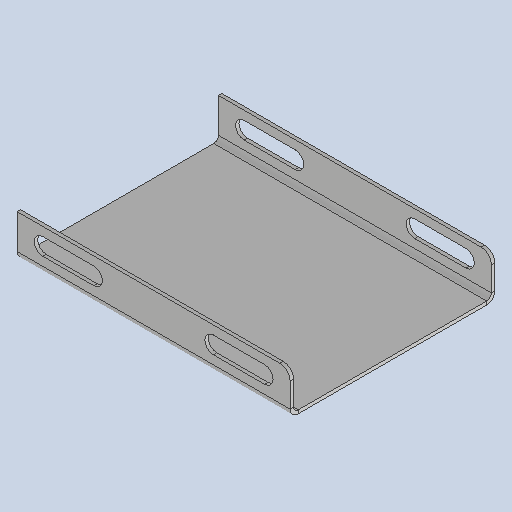
# Autodesk Inventor part: TRM 026 right board damper
Saved by Autodesk Inventor 2025 (Build 290162010, 162A)
## iProperties
Created: 2024-08-07
Part Number: TRM 026 right board damper
Material: AISI 304
Document SubType Name: Sheet Metal
Designer: pokla
Density: 8.02768 g/cm^3
Flat Pattern Width: 16.2404 cm
Flat Pattern Length: 16 cm
Flat Pattern Area: 259.846 cm^2
Sheet Metal Rule: AISI304 2mm Die16
Sheet Metal Width: 162.404 mm
Sheet Metal Length: 160.000 mm
Sheet Metal Area: 25984.637 mm^2
Appearance: Default
Stock Number: ТРМ 026 правый борт успокоитель
Mass: 393.603 g
Surface Area: 510.428 cm^2
Volume: 49.0307 cm^3
Author: pokla
Autodesk Inventor part; units mm, degrees
note: some values were not read from the file. Chosen so that the rebuilt part matches the saved one: flange form of "Plate2".
ref_plane "YZ Plane" through (0, 0, 0) normal (1, 0, 0) x (0, 1, 0)
ref_plane "XZ Plane" through (0, 0, 0) normal (0, 1, 0) x (-1, 0, 0)
ref_plane "XY Plane" through (0, 0, 0) normal (0, 0, 1) x (1, 0, 0)
sketch "Sketch1" plane through (0, 0, 0) normal (0, 0, 1) x (1, 0, 0)
  line L0 (-80, -60) -> (80, -60)
  line L1 (80, -60) -> (80, 60)
  line L2 (80, 60) -> (-80, 60)
  line L3 (-80, 60) -> (-80, -60)
  line L4 (-80, -60) -> (80, 60) construction
  line L5 (80, -60) -> (-80, 60) construction
  point P0 (0, 0)
  dimension "d0" = 160
  dimension "d1" = 120
  measures "d0" distance of L2.end L1.end
  measures "d1" distance of L1.end L0.end
extrude "Plate1" add sketch "Sketch1" along normal blind 2
sketch "Sketch2" plane through (0, 0, 0) normal (0, 0, -1) x (-1, 0, 0)
  line L0 (-60, 40) -> (140, 40) construction
  line L1 (140, 40) -> (140, 20) construction
  line L2 (140, 20) -> (-60, 20) construction
  line L3 (-60, 20) -> (-60, 40) construction
  line L4 (-80, 60) -> (80, 60) projected
  line L5 (-80, -60) -> (-80, 60) projected
  point P0 (0, 0)
  point P1 (-48, 100)
  point P2 (-50, 98)
  dimension "d6" = 200
  dimension "d9" = 20
  dimension "d10" = 20
  dimension "d11" = 20
  constraints: 4 other
  measures "d6" distance of L0.start L0.end
  measures "d9" distance of L0.end L1.end
  measures "d11" length of L3
mark "Mark1"
sketch "Sketch3" plane through (80, 58, 0) normal (0, 1, 0) x (-1, 0, 0)
  line L0 (160, 0) -> (0, 0)
  line L1 (0, 0) -> (0, -25)
  line L2 (0, -25) -> (160, -25)
  line L3 (160, -25) -> (160, 0)
  constraints: 6 end point, 1 horizontal, 1 perpendicular, 1 vertical
edge flange "Flange1" height 25 angle 90 thickness 2 bend radius 2.75 thickness toward (0, 1, 0) relief round relief width 2 relief depth 1 corner gap 2.75 corner form 0 edges at (0, 60, 0) (0, -60, 0) wall of the first edge with corners at (-80, 58, 0) (80, 58, 0) (80, 58, 25) (-80, 58, 25)
bend "Bend1"
corner "Corner1"
sketch "Sketch4" plane through (0, 0, 0) normal (0, 1, 0) x (-1, 0, 0)
  line L0 (-80, 4.75) -> (80, 4.75) construction
  line L1 (80, 4.75) -> (80, 25) projected
  line L2 (80, 25) -> (-80, 25) construction
  line L3 (-80, 4.75) -> (-80, 25) projected
  line L4 (-65, 14.875) -> (-35, 14.875) construction
  line L5 (-65, 9.875) -> (-35, 9.875)
  line L6 (-35, 19.875) -> (-65, 19.875)
  arc A0 (-65, 19.875) -> (-65, 9.875) centre (-65, 14.875) ccw
  arc A1 (-35, 9.875) -> (-35, 19.875) centre (-35, 14.875) ccw
  line L7 (35, 14.875) -> (65, 14.875) construction
  line L8 (35, 9.875) -> (65, 9.875)
  line L9 (65, 19.875) -> (35, 19.875)
  arc A2 (35, 19.875) -> (35, 9.875) centre (35, 14.875) ccw
  arc A3 (65, 9.875) -> (65, 19.875) centre (65, 14.875) ccw
  line L10 (0, 4.75) -> (0, 25) construction
  point P0 (0, 0)
  point P1 (-50, 14.875)
  point P2 (50, 14.875)
  point P3 (-80, 14.875)
  dimension "d22" = 30
  dimension "d23" = 10
  dimension "d24" = 100
  constraints: 18 end point, 8 point on circle, 8 tangent, 5 midpoint, 4 centre point, 3 parallel, 2 point on line, 1 collinear, 1 equal radius, 1 horizontal alignment, 1 symmetric about line, 1 other
  measures "d22" distance of L4.start L4.end
  measures "d23" diameter of A1
  measures "d24" distance of point (50, 14.875) point (-50, 14.875)
extrude "Extrusion1" cut sketch "Sketch4" along normal through all both and the other way through all
fillet "Corner Round1" radius 6 2 edges at (80, 59, 25) (80, -59, 25)
equation "\"d2\" = Thickness"
equation "\"d12\" = BendReliefWidth"
equation "\"d13\" = BendReliefDepth"
equation "\"d14\" = MinimumRemnant"
equation "\"d15\" = TransitionRadius"
equation "\"d18\" = BendRadius"
equation "\"d19\" = CornerReliefSize"
equation "\"d20\" = GapSize"
equation "\"d21\" = JacobiRadiusSize"
equation "\"BendReliefWidth\" = Thickness"
equation "\"BendReliefDepth\" = 0.5 * Thickness"
equation "\"CornerReliefSize\" = 4 * Thickness"
equation "\"MinimumRemnant\" = 2 * Thickness"
equation "\"TransitionRadius\" = BendRadius"
equation "\"JacobiRadiusSize\" = BendRadius"
equation "\"GapSize\" = Thickness"
equation "\"Thickness\" = 2"
equation "\"BendRadius\" = 2.75"
body "Solid1"
